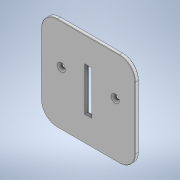
# Autodesk Inventor part: TopV3Back
Saved by Autodesk Inventor 2021 (Build 250183000, 183)
## iProperties
Created: 2021-02-17
Part Number: TopV3Back
Material: Generic
Document SubType Name: Modeling
Designer: Viktor
Density: 1 g/cm^3
Appearance: Default
Author: Viktor
Autodesk Inventor part; units mm, degrees
ref_plane "YZ Plane" through (0, 0, 0) normal (1, 0, 0) x (0, 1, 0)
ref_plane "XZ Plane" through (0, 0, 0) normal (0, 1, 0) x (-1, 0, 0)
ref_plane "XY Plane" through (0, 0, 0) normal (0, 0, 1) x (1, 0, 0)
sketch "Sketch1" plane through (0, 0, 0) normal (0, 0, 1) x (1, 0, 0)
  line L0 (-40, -40) -> (40, -40)
  line L1 (40, -40) -> (40, 40)
  line L2 (40, 40) -> (-40, 40)
  line L3 (-40, 40) -> (-40, -40)
  line L4 (-40, -40) -> (40, 40) construction
  line L5 (40, -40) -> (-40, 40) construction
  line L6 (-2.8, -18.3) -> (2.8, -18.3)
  line L7 (2.8, -18.3) -> (2.8, 18.3)
  line L8 (2.8, 18.3) -> (-2.8, 18.3)
  line L9 (-2.8, 18.3) -> (-2.8, -18.3)
  line L10 (-2.8, -18.3) -> (2.8, 18.3) construction
  line L11 (2.8, -18.3) -> (-2.8, 18.3) construction
  circle A0 centre (23, 6) radius 1.8
  line L12 (0, 56) -> (0, -56) construction
  circle A1 centre (-23, 6) radius 1.8
  point P0 (0, 0)
  dimension "d0" = 80
  dimension "d1" = 80
  dimension "d2" = 5.6
  dimension "d3" = 36.6
  dimension "d4" = 3.6
  dimension "d5" = 12.3
  dimension "d6" = 23
  constraints: 24 end point, 4 midpoint, 4 parallel, 2 centre point, 2 horizontal, 2 perpendicular, 1 symmetric about line, 1 other
  measures "d0" distance between parallel lines of L1 L3
  measures "d1" distance between parallel lines of L0 L2
  measures "d2" distance between parallel lines of L7 L9
  measures "d3" distance between parallel lines of L6 L8
  measures "d4" diameter of A0
  measures "d5" distance from line of L8 A0.centre
  measures "d6" horizontal distance of point (0, 0) A0.centre
extrude "Extrusion1" add sketch "Sketch1" along normal blind 3
fillet "Fillet1" radius 13.5 4 edges at (40, 40, 1.5) (40, -40, 1.5) (-40, -40, 1.5) (-40, 40, 1.5)
chamfer "Chamfer1" distance 1.7 angle 45 2 edges at (-24.8, 6, 3) (21.2, 6, 3)
chamfer "Chamfer2" distance 0.3 angle 45 25 edges at (-40, 0, 0) (-36.0459, -36.0459, 0) (0, -40, 0) (36.0459, -36.0459, 0) (40, 0, 0) (36.0459, 36.0459, 0) (0, 40, 0) (-36.0459, 36.0459, 0) (-40, 0, 3) (-36.0459, -36.0459, 3) (0, -40, 3) (36.0459, -36.0459, 3) (40, 0, 3) (36.0459, 36.0459, 3) (0, 40, 3) (-36.0459, 36.0459, 3) (-2.8, 0, 3) (2.8, 0, 3) (0, 18.3, 3) (2.8, 0, 0) (0, -18.3, 3) (0, 18.3, 0) (0, -18.3, 0) (-24.8, 6, 0) (21.2, 6, 0)
body "Solid1"
